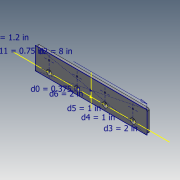
# Autodesk Inventor part: VP HINGE SHIFT PLATE
Saved by Autodesk Inventor 2018.3 (Build 223284000, 284)
## iProperties
Created: 2019-10-29
Material: Generic
Vendor: HHMI: JRC - ID&F
Document SubType Name: Modeling
Designer: arnoldj
Density: 1 g/cm^3
Appearance: Default
RuleStatus: InUse
AfterDocSave0: file://Part Number Cleaner
DESIGN DEPARTMENT: HHMI: JRC - ID&F
ALTERED ITEM PART NUMBER: N/A
ALTERED ITEM VENDOR: N/A
ALTERED ITEM DESCRIPTION: N/A
Author: arnoldj
Revision Number: 0
Autodesk Inventor part; units mm, degrees
ref_plane "YZ Plane" through (0, 0, 0) normal (1, 0, 0) x (0, 1, 0)
ref_plane "XZ Plane" through (0, 0, 0) normal (0, 1, 0) x (-1, 0, 0)
ref_plane "XY Plane" through (0, 0, 0) normal (0, 0, 1) x (1, 0, 0)
sketch "Sketch1" plane through (0, 0, 0) normal (0, 0, 1) x (1, 0, 0)
  line L0 (0, 38.481) -> (0, -17.526) projected
  line L1 (-142.24, 0) -> (142.24, 0) projected
  line L2 (101.6, 30.48) -> (-101.6, 30.48)
  line L3 (-101.6, 30.48) -> (-101.6, -9.525)
  line L4 (-101.6, -9.525) -> (101.6, -9.525)
  line L5 (101.6, -9.525) -> (101.6, 30.48)
  line L6 (101.6, 30.48) -> (-101.6, -9.525) construction
  line L7 (-101.6, 30.48) -> (101.6, -9.525) construction
  point P0 (0, 0)
  point P1 (0, 10.4775)
  point P2 (-76.2, 0)
  point P3 (-25.4, 0)
  point P4 (25.4, 0)
  point P5 (76.2, 0)
  point P6 (-76.2, 19.05)
  point P7 (-25.4, 19.05)
  point P8 (25.4, 19.05)
  point P9 (76.2, 19.05)
  dimension "d0" = 9.525
  dimension "d1" = 30.48
  dimension "d2" = 203.2
  dimension "d3" = 50.8
  dimension "d4" = 25.4
  dimension "d5" = 25.4
  dimension "d6" = 50.8
  dimension "d11" = 19.05
  constraints: 12 end point, 4 point on line, 3 midpoint, 2 parallel, 1 horizontal, 1 perpendicular, 1 vertical, 4 other
  measures "d0" distance between parallel lines of L4 L1
  measures "d1" distance between parallel lines of L1 L2
  measures "d2" distance of L2.start L2.end
  measures "d3" distance of point (25.4, 0) point (76.2, 0)
  measures "d4" distance from line of point (25.4, 0) L0
  measures "d5" distance from line of L0 point (-25.4, 0)
  measures "d6" distance of point (-25.4, 0) point (-76.2, 0)
  measures "d11" distance of point (-76.2, 0) point (-76.2, 19.05)
extrude "Extrusion1" add sketch "Sketch1" against normal blind 4.4958
hole "Hole1" at (-76.2, 0, 0) at (-25.4, 0, 0) at (25.4, 0, 0) at (76.2, 0, 0) direction (0, 0, -1) diameter 4.4958 end through all countersink diameter 9.398 countersink angle 90 clearance for "Flat Head Machine Screw" size "M4" standard "Ansi Metric M Profile"
hole "Hole2" at (-76.2, 19.05, 0) at (-25.4, 19.05, 0) at (25.4, 19.05, 0) at (76.2, 19.05, 0) direction (0, 0, -1) diameter 3.1242 end through all
fillet "Fillet1" radius 3.175 4 edges at (-101.6, 30.48, -2.2479) (101.6, 30.48, -2.2479) (101.6, -9.525, -2.2479) (-101.6, -9.525, -2.2479)
body "Solid1"
